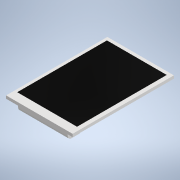
# Autodesk Inventor part: Display
Saved by Autodesk Inventor 2022 (Build 260153000, 153)
## iProperties
Created: 2020-11-26
Part Number: Display
Material: Generic
Document SubType Name: Modeling
Designer: simen
Density: 1 g/cm^3
Appearance: Default
Author: simen
Autodesk Inventor part; units mm, degrees
ref_plane "YZ Plane" through (0, 0, 0) normal (1, 0, 0) x (0, 1, 0)
ref_plane "XZ Plane" through (0, 0, 0) normal (0, 1, 0) x (-1, 0, 0)
ref_plane "XY Plane" through (0, 0, 0) normal (0, 0, 1) x (1, 0, 0)
sketch "Sketch1" plane through (0, 0, 0) normal (0, 1, 0) x (-1, 0, 0)
  line L0 (42.2226, 53.0438) -> (-12.2774, 53.0438)
  line L1 (-12.2774, 53.0438) -> (-12.2774, -29.9562)
  line L2 (-12.2774, -29.9562) -> (42.2226, -29.9562)
  line L3 (42.2226, -29.9562) -> (42.2226, 53.0438)
  point P0 (0, 0)
  dimension "d0" = 54.5
  dimension "d1" = 83
  constraints: 8 end point, 2 parallel, 1 horizontal, 1 perpendicular
  measures "d0" distance of L2.end L1.end
  measures "d1" distance of L1.end L0.end
extrude "Extrusion1" add sketch "Sketch1" along normal blind 2.35
sketch "Sketch2" plane through (0, 2.35, 0) normal (0, 1, 0) x (1, 0, 0)
  line L0 (-39.8226, -46.2538) -> (9.1374, -46.2538)
  line L1 (9.1374, -46.2538) -> (9.1374, 27.1862)
  line L2 (9.1374, 27.1862) -> (-39.8226, 27.1862)
  line L3 (-39.8226, 27.1862) -> (-39.8226, -46.2538)
  line L4 (12.2774, -53.0438) -> (12.2774, 29.9562) projected
  line L5 (12.2774, 29.9562) -> (-42.2226, 29.9562) projected
  line L6 (-42.2226, 29.9562) -> (-42.2226, -53.0438) projected
  line L7 (-42.2226, -53.0438) -> (12.2774, -53.0438) projected
  point P0 (0, 0)
  dimension "d4" = 48.96
  dimension "d5" = 73.44
  dimension "d6" = 2.77
  dimension "d7" = 2.4
  constraints: 8 end point, 2 parallel, 1 horizontal, 1 perpendicular
  measures "d4" distance of L2.end L1.end
  measures "d5" distance of L1.end L0.end
  measures "d6" distance between parallel lines of L5 L2
  measures "d7" distance between parallel lines of L6 L3
extrude "Extrusion2" add sketch "Sketch2" along normal blind 0.1 contours L3 L2 L1 L0
sketch "Sketch3" plane through (0, 0, 0) normal (0, -1, 0) x (1, 0, 0)
  line L0 (12.2774, 53.0438) -> (12.2774, -29.9562) projected
  line L1 (-42.2226, 53.0438) -> (12.2774, 53.0438) projected
  line L2 (-42.2226, -29.9562) -> (-42.2226, 53.0438) projected
  line L3 (12.2774, -29.9562) -> (-42.2226, -29.9562) projected
  line L4 (-42.2226, 53.0438) -> (12.2774, 53.0438) projected
  line L5 (-32.3226, 53.0438) -> (-32.3226, 31.8438)
  line L6 (-32.3226, 31.8438) -> (-11.8226, 31.8438)
  line L7 (-11.8226, 31.8438) -> (-11.8226, 43.0438)
  line L8 (-11.8226, 43.0438) -> (8.2974, 43.0438)
  line L9 (8.2974, 43.0438) -> (8.2974, 53.0438)
  point P0 (0, 0)
  dimension "d11" = 9.9
  dimension "d12" = 21.2
  dimension "d13" = 3.98
  dimension "d14" = 20.5
  dimension "d15" = 10
  constraints: 10 end point, 4 perpendicular, 2 point on line, 1 horizontal
  measures "d11" distance between parallel lines of L2 L5
  measures "d12" distance of L5.start L5.end
  measures "d13" distance between parallel lines of L0 L9
  measures "d14" distance of L5.end L6.end
  measures "d15" distance between parallel lines of L1 L8
extrude "Extrusion3" add sketch "Sketch3" along normal blind 4.3 contours L9 L8 L7 L6 L5 L1
fillet "Fillet2" radius 3 1 edges at (-12.0126, -4.3, 53.0438)
sketch "Sketch4" plane through (-11.8226, 0, 31.8438) normal (0, 0, -1) x (-1, 0, 0)
  line L0 (0, 0) -> (20.5, 0) projected
  line L1 (0, 0) -> (0, -4.3) projected
  line L2 (20.5, -4.3) -> (0, -4.3) projected
  line L3 (20.5, 0) -> (20.5, -4.3) projected
  line L4 (0, -2.3) -> (20.5, -2.3)
  line L5 (20.5, -1.3) -> (20.5, -4.3) projected
  point P0 (-11.8226, 0)
  point P1 (0, -2.3)
  dimension "d19" = 2
  constraints: 2 end point, 1 perpendicular, 1 point on line
  measures "d19" distance between parallel lines of L2 L4
extrude "Extrusion4" cut sketch "Sketch4" against normal blind 3.5 contours L4 L3 L2 L1
body "Solid1"
